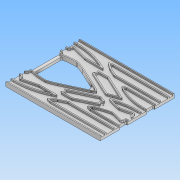
# Autodesk Inventor part: PocketPoint
Saved by Autodesk Inventor 2021 (Build 250183000, 183)
## iProperties
Created: 2021-03-04
Part Number: PocketPoint
Material: 一般
Document SubType Name: Modeling
Designer: kumagai
Density: 1 g/cm^3
Appearance: 既定
Author: kumagai
Autodesk Inventor part; units mm, degrees
ref_plane "YZ Plane" through (0, 0, 0) normal (1, 0, 0) x (0, 1, 0)
ref_plane "XZ Plane" through (0, 0, 0) normal (0, 1, 0) x (-1, 0, 0)
ref_plane "XY Plane" through (0, 0, 0) normal (0, 0, 1) x (1, 0, 0)
sketch "スケッチ1" plane through (0, 0, 0) normal (0, 1, 0) x (-1, 0, 0)
  line L0 (0, -199.2237) -> (0, 200.4653) projected
  line L1 (-205.9572, 0) -> (190.052, 0) projected
  line L2 (92.5, -106.7983) -> (92.5, -71.9832)
  line L3 (-92.5, -104.7638) -> (-92.5, -76.5833)
  line L4 (-113.8272, -72.75) -> (-139.8678, -72.75)
  line L5 (-115.1264, 72.75) -> (-146.0495, 72.75)
  line L6 (-92.5, -72.75) -> (92.5, -72.75)
  line L7 (92.5, -72.75) -> (92.5, -34.75)
  line L8 (-92.5, -34.75) -> (-92.5, -72.75)
  line L9 (-92.5, 72.75) -> (92.5, 72.75)
  line L10 (92.5, 72.75) -> (92.5, 34.75)
  line L11 (-92.5, 34.75) -> (-92.5, 72.75)
  line L12 (128.5967, -53.75) -> (-115.1264, -53.75)
  line L13 (133.4793, 53.75) -> (-123.0769, 53.75)
  line L14 (-117.8804, 0) -> (-149.3845, 0)
  line L15 (92.5, -70.75) -> (-92.5, -70.75)
  line L16 (92.5, 70.75) -> (-92.5, 70.75)
  line L17 (-92.5, -19) -> (-92.5, 19)
  line L18 (-92.5, 19) -> (-90.5855, 19)
  line L19 (-92.5, -19) -> (-87.5, -19)
  line L20 (-92.5, -17) -> (-87.5, -17)
  line L21 (-92.5, 17) -> (-90.5855, 17)
  line L22 (92.5, -63.05) -> (-92.5, -63.05)
  line L23 (92.5, -60.65) -> (-92.5, -60.65)
  line L24 (92.5, -46.85) -> (-92.5, -46.85)
  line L25 (92.5, -44.45) -> (-92.5, -44.45)
  line L26 (-111.5116, -25.1237) -> (108.8826, 77.6478)
  line L27 (-111.5116, 25.1237) -> (108.8826, -77.6478)
  line L28 (-97.9488, -37.5567) -> (-102.497, -39.6775)
  line L29 (-102.6652, -28.6119) -> (-107.2133, -30.7327)
  line L30 (-101.0738, -30.5179) -> (-105.622, -32.6387)
  line L31 (-96.3211, -39.0044) -> (-100.8692, -41.1253)
  line L32 (-108.7666, -16.2304) -> (-113.3147, -18.3512)
  line L33 (-110.4448, -14.3649) -> (-114.993, -16.4857)
  line L34 (-114.1016, -7.574) -> (-118.6498, -9.6949)
  line L35 (-114.2638, -5.4429) -> (-118.8119, -7.5637)
  line L36 (-97.9488, 37.5567) -> (-102.497, 39.6775)
  line L37 (-102.6652, 28.6119) -> (-107.2133, 30.7327)
  line L38 (-101.0738, 30.5179) -> (-105.622, 32.6387)
  line L39 (-96.3211, 39.0044) -> (-100.8692, 41.1253)
  line L40 (-108.7666, 16.2304) -> (-113.3147, 18.3512)
  line L41 (-110.4448, 14.3649) -> (-114.993, 16.4857)
  line L42 (-114.1016, 7.574) -> (-118.6498, 9.6949)
  line L43 (-114.2638, 5.4429) -> (-118.8119, 7.5637)
  line L44 (-5.3544, 3.414) -> (38.5952, 23.9081)
  line L45 (-6.1996, 5.2266) -> (37.75, 25.7207)
  arc A0 (54.8664, 32.1363) -> (37.75, 25.7207) centre (87.5, -80.9685) ccw
  arc A1 (87.5, 60.65) -> (27.6494, 47.3814) centre (87.5, -80.9685) ccw
  arc A2 (87.5, 63.05) -> (26.6351, 49.5566) centre (87.5, -80.9685) ccw
  line L46 (87.5, -11.0193) -> (87.5, 9.6949)
  line L47 (22.0715, 26.9057) -> (-24.3751, 5.2473)
  arc A3 (20.6744, 35.131) -> (22.099, 28.705) centre (24.0122, 32.5) ccw
  line L48 (19.005, 28.1239) -> (-25.3894, 7.4224)
  line L49 (92.5, 34.75) -> (91.5, 34.75)
  arc A4 (17.6247, 34.35) -> (19.005, 28.1239) centre (24.0122, 32.5) ccw
  line L50 (11.7288, 51.1017) -> (-1.4507, 44.9559)
  line L51 (10.7146, 53.2768) -> (-2.465, 47.1311)
  line L52 (-3.7329, 46.85) -> (-92.5, 46.85)
  line L53 (-3.7329, 44.45) -> (-92.5, 44.45)
  line L54 (12.544, 51.5723) -> (23.6088, 59.32)
  line L55 (23.294, 61.105) -> (16.7221, 62.866)
  line L56 (11.1674, 53.5383) -> (19.7729, 59.5639)
  line L57 (92.5, 60.65) -> (87.5, 60.65)
  line L58 (15.3244, 60.65) -> (-92.5, 60.65)
  line L59 (92.5, 63.05) -> (87.5, 63.05)
  line L60 (15.3244, 63.05) -> (-92.5, 63.05)
  line L61 (19.7729, 59.5639) -> (16.1009, 60.5478)
  arc A5 (23.6088, 59.32) -> (23.294, 61.105) centre (23.0352, 60.1391) ccw
  arc A6 (10.7146, 53.2768) -> (11.1674, 53.5383) centre (9.4467, 55.9957) ccw
  arc A7 (16.1009, 60.5478) -> (15.3244, 60.65) centre (15.3244, 57.65) ccw
  arc A8 (11.7288, 51.1017) -> (12.544, 51.5723) centre (9.4467, 55.9957) ccw
  arc A9 (16.7221, 62.866) -> (15.3244, 63.05) centre (15.3244, 57.65) ccw
  arc A10 (-3.7329, 44.45) -> (-1.4507, 44.9559) centre (-3.7329, 49.85) ccw
  arc A11 (-3.7329, 46.85) -> (-2.465, 47.1311) centre (-3.7329, 49.85) ccw
  line L62 (-35.4314, 29.1105) -> (-37.75, 28.0293)
  line L63 (-36.2766, 30.9231) -> (-38.5952, 29.8419)
  line L64 (-37.9474, 36.75) -> (-87.5, 36.75)
  line L65 (17.6247, 34.35) -> (0.3685, 34.35)
  line L66 (-37.9474, 34.75) -> (-87.5, 34.75)
  arc A12 (-63.697, 21.4746) -> (-38.5952, 29.8419) centre (-87.5, 134.7185) ccw
  arc A13 (-63.2856, 19.5173) -> (-37.75, 28.0293) centre (-87.5, 134.7185) ccw
  line L67 (-87.5, 126.6079) -> (-87.5, 142.8291)
  line L68 (26.5097, 46.85) -> (27.6494, 47.3814)
  line L69 (-38.0005, 19.4165) -> (-1.9137, 36.2441)
  line L70 (19.7721, 46.3563) -> (26.6351, 49.5566)
  line L71 (85.7327, 47.3926) -> (84.7595, 51.2358)
  line L72 (83.5446, 51.9597) -> (54.5417, 44.6152)
  line L73 (88.0593, 47.9818) -> (87.086, 51.825)
  line L74 (82.9554, 54.2863) -> (53.9526, 46.9418)
  line L75 (92.5, 46.85) -> (89.5134, 46.85)
  line L76 (53.2161, 46.85) -> (26.5097, 46.85)
  line L77 (92.5, 44.45) -> (89.5134, 44.45)
  line L78 (53.2161, 44.45) -> (20.1947, 44.45)
  line L79 (92.5, 36.75) -> (91.5, 36.75)
  line L80 (19.8891, 36.75) -> (0.3685, 36.75)
  circle A14 centre (24.0122, 32.5) radius 1
  arc A15 (22.0715, 26.9057) -> (22.099, 28.705) centre (21.6489, 27.812) ccw
  arc A16 (20.6744, 35.131) -> (19.8891, 36.75) centre (19.8891, 35.75) ccw
  arc A17 (62.91, 42.0158) -> (40.2524, 35.2101) centre (87.5, -80.9685) ccw
  line L81 (87.5, 32.75) -> (87.5, 30.0175)
  arc A18 (86.2722, 29.0437) -> (56.1923, 32.3319) centre (57.7026, -93.0817) ccw
  arc A19 (85.8166, 27.0963) -> (56.2163, 30.332) centre (57.7026, -93.0817) ccw
  arc A20 (55.4208, 30.2147) -> (38.5952, 23.9081) centre (87.5, -80.9685) ccw
  arc A21 (88.0593, 47.9818) -> (89.5134, 46.85) centre (89.5134, 48.35) ccw
  arc A22 (84.7595, 51.2358) -> (83.5446, 51.9597) centre (83.7901, 50.9903) ccw
  arc A23 (85.7327, 47.3926) -> (89.5134, 44.45) centre (89.5134, 48.35) ccw
  arc A24 (87.086, 51.825) -> (82.9554, 54.2863) centre (83.7901, 50.9903) ccw
  arc A25 (53.2161, 44.45) -> (54.5417, 44.6152) centre (53.2161, 49.85) ccw
  arc A26 (53.2161, 46.85) -> (53.9526, 46.9418) centre (53.2161, 49.85) ccw
  arc A27 (19.7721, 46.3563) -> (20.1947, 44.45) centre (20.1947, 45.45) ccw
  arc A28 (91.5, 34.75) -> (89.5, 32.75) centre (91.5, 32.75) ccw
  arc A29 (91.5, 36.75) -> (87.5, 32.75) centre (91.5, 32.75) ccw
  line L82 (89.5, 32.75) -> (89.5, 30.0175)
  arc A30 (86.2722, 29.0437) -> (87.5, 30.0175) centre (86.5, 30.0175) ccw
  arc A31 (85.8166, 27.0963) -> (89.5, 30.0175) centre (86.5, 30.0175) ccw
  arc A32 (56.2163, 30.332) -> (55.4208, 30.2147) centre (56.2525, 27.3322) ccw
  arc A33 (56.1923, 32.3319) -> (54.8664, 32.1363) centre (56.2525, 27.3322) ccw
  line L83 (-34.6766, 29.5463) -> (-29.7157, 33.02)
  line L84 (-30.0304, 34.805) -> (-36.6533, 36.5796)
  line L85 (-35.8238, 31.1846) -> (-32.6195, 33.4282)
  line L86 (-32.6195, 33.4282) -> (-37.1709, 34.6478)
  arc A34 (-36.2766, 30.9231) -> (-35.8238, 31.1846) centre (-37.5445, 33.642) ccw
  arc A35 (-35.4314, 29.1105) -> (-34.6766, 29.5463) centre (-37.5445, 33.642) ccw
  line L87 (-87.5, 36.75) -> (-92.5, 36.75)
  arc A36 (-36.6533, 36.5796) -> (-37.9474, 36.75) centre (-37.9474, 31.75) ccw
  line L88 (-87.5, 34.75) -> (-92.5, 34.75)
  arc A37 (-37.1709, 34.6478) -> (-37.9474, 34.75) centre (-37.9474, 31.75) ccw
  arc A38 (-29.7157, 33.02) -> (-30.0304, 34.805) centre (-30.2892, 33.8391) ccw
  line L89 (24.6013, -19.5893) -> (0, -8.1176)
  line L90 (22.0715, -26.9057) -> (-24.3751, -5.2473)
  line L91 (19.005, -28.1239) -> (-25.3894, -7.4224)
  arc A39 (-39.1516, 0.942) -> (-62.6685, 7.1431) centre (-87.5, -134.7185) ccw
  arc A40 (-87.5, -6.9) -> (-43.8339, 0) centre (-87.5, 134.7185) ccw
  arc A41 (-117.0028, -6.2788) -> (-116.3471, -6.4144) centre (-87.5, 134.7185) ccw
  line L92 (-92.5, -9.3) -> (-87.5, -9.3)
  line L93 (-92.5, -6.9) -> (-87.5, -6.9)
  arc A42 (-87.5, -9.3) -> (-39.1516, -0.942) centre (-87.5, 134.7185) ccw
  line L94 (-92.5, 6.9) -> (-90.4054, 6.9)
  line L95 (-92.5, 9.3) -> (-90.4054, 9.3)
  arc A43 (-28.7483, 5.1627) -> (-37.3938, 8.4872) centre (-87.5, -134.7185) ccw
  arc A44 (-37.6117, 10.2675) -> (-38.028, 17.6172) centre (-39.9412, 13.8222) ccw
  arc A45 (-34.4994, 10) -> (-34.934, 18.1983) centre (-39.9412, 13.8222) ccw
  line L96 (20.097, -15.2822) -> (0, -5.9108)
  arc A46 (22.099, -28.705) -> (20.6744, -35.131) centre (24.0122, -32.5) ccw
  arc A47 (19.005, -28.1239) -> (17.6247, -34.35) centre (24.0122, -32.5) ccw
  circle A48 centre (24.0122, -32.5) radius 1
  arc A49 (22.099, -28.705) -> (22.0715, -26.9057) centre (21.6489, -27.812) ccw
  arc A50 (19.8891, -36.75) -> (20.6744, -35.131) centre (19.8891, -35.75) ccw
  line L97 (92.5, -36.75) -> (42.3385, -36.75)
  line L98 (92.5, -34.75) -> (42.3385, -34.75)
  line L99 (-78.1824, -36.75) -> (-92.5, -36.75)
  line L100 (-78.1824, -34.75) -> (-92.5, -34.75)
  arc A51 (0.3685, 34.35) -> (-0.8994, 34.0689) centre (0.3685, 31.35) ccw
  arc A52 (0.3685, 36.75) -> (-1.9137, 36.2441) centre (0.3685, 31.35) ccw
  line L101 (-35.4314, -29.1105) -> (-37.75, -28.0293)
  line L102 (-36.2766, -30.9231) -> (-38.5952, -29.8419)
  line L103 (-37.9474, -36.75) -> (-87.5, -36.75)
  line L104 (17.6247, -34.35) -> (0.3685, -34.35)
  line L105 (-37.9474, -34.75) -> (-87.5, -34.75)
  line L106 (19.8891, -36.75) -> (0.3685, -36.75)
  line L107 (-34.6766, -29.5463) -> (-29.7157, -33.02)
  line L108 (-30.0304, -34.805) -> (-36.6533, -36.5796)
  line L109 (-35.8238, -31.1846) -> (-32.6195, -33.4282)
  line L110 (-32.6195, -33.4282) -> (-37.1709, -34.6478)
  arc A53 (-35.8238, -31.1846) -> (-36.2766, -30.9231) centre (-37.5445, -33.642) ccw
  arc A54 (-34.6766, -29.5463) -> (-35.4314, -29.1105) centre (-37.5445, -33.642) ccw
  arc A55 (-37.9474, -36.75) -> (-36.6533, -36.5796) centre (-37.9474, -31.75) ccw
  arc A56 (-37.9474, -34.75) -> (-37.1709, -34.6478) centre (-37.9474, -31.75) ccw
  arc A57 (-30.0304, -34.805) -> (-29.7157, -33.02) centre (-30.2892, -33.8391) ccw
  arc A58 (-0.8994, -34.0689) -> (0.3685, -34.35) centre (0.3685, -31.35) ccw
  arc A59 (-1.9137, -36.2441) -> (0.3685, -36.75) centre (0.3685, -31.35) ccw
  arc A60 (-38.5952, -29.8419) -> (-87.5, -19) centre (-87.5, -134.7185) ccw
  arc A61 (-37.75, -28.0293) -> (-87.5, -17) centre (-87.5, -134.7185) ccw
  arc A62 (-36.065, -8.0153) -> (-28.7483, -5.1627) centre (-87.5, 134.7185) ccw
  line L111 (-1.9137, -36.2441) -> (-48.7506, -14.4036)
  line L112 (-0.8994, -34.0689) -> (-44.6592, -13.6634)
  arc A63 (-35.2514, -10.2732) -> (-27.8189, -7.3754) centre (-87.5, 134.7185) ccw
  arc A64 (-48.667, -12.5565) -> (-48.7506, -14.4036) centre (-48.328, -13.4973) ccw
  arc A65 (-25.3894, -7.4224) -> (-27.8189, -7.3754) centre (-26.6572, -10.1414) ccw
  arc A66 (-24.3751, -5.2473) -> (-28.7483, -5.1627) centre (-26.6572, -10.1414) ccw
  arc A67 (-28.7483, 5.1627) -> (-24.3751, 5.2473) centre (-26.6572, 10.1414) ccw
  line L113 (-34.934, 18.1983) -> (-0.8994, 34.0689)
  arc A68 (-37.6117, 10.2675) -> (-37.3938, 8.4872) centre (-37.0635, 9.4311) ccw
  arc A69 (-38.0005, 19.4165) -> (-38.028, 17.6172) centre (-37.5779, 18.5102) ccw
  arc A70 (-27.8189, 7.3754) -> (-34.4994, 10) centre (-87.5, -134.7185) ccw
  arc A71 (-27.8189, 7.3754) -> (-25.3894, 7.4224) centre (-26.6572, 10.1414) ccw
  arc A72 (-52.3064, 12.8617) -> (-70.3129, 16.0234) centre (-87.5, -134.7185) ccw
  arc A73 (-74.1443, 10.0131) -> (-58.4543, 12.7097) centre (-87.5, 134.7185) ccw
  line L114 (-87.4523, 6.8287) -> (-86.6895, 2.5679)
  line L115 (-39.9412, 13.8222) -> (-87.1898, 5.3626)
  line L116 (-86.992, 23.7251) -> (-87.6188, 19.5542)
  line L117 (-39.9412, 13.8222) -> (-87.4082, 20.9556)
  arc A74 (-64.5674, 7.1366) -> (-85.3887, 1.7956) centre (-37.375, -142.1252) ccw
  arc A75 (-85.6835, 24.524) -> (-65.0909, 19.4711) centre (-45.6063, 143.3669) ccw
  line L118 (-89.8148, 6.4057) -> (-89.0519, 2.145)
  arc A76 (-89.8148, 6.4057) -> (-90.4054, 6.9) centre (-90.4054, 6.3) ccw
  arc A77 (-87.4523, 6.8287) -> (-90.4054, 9.3) centre (-90.4054, 6.3) ccw
  arc A78 (-86.6895, 2.5679) -> (-85.3887, 1.7956) centre (-85.7051, 2.7442) ccw
  arc A79 (-89.0519, 2.145) -> (-84.6292, -0.4811) centre (-85.7051, 2.7442) ccw
  arc A80 (-64.1372, 4.7754) -> (-84.6292, -0.4811) centre (-37.375, -142.1252) ccw
  arc A81 (-43.8339, 0) -> (-63.0823, 4.7791) centre (-87.5, -134.7185) ccw
  arc A82 (-62.6685, 7.1431) -> (-64.5674, 7.1366) centre (-63.5996, 1.824) ccw
  arc A83 (-63.0823, 4.7791) -> (-64.1372, 4.7754) centre (-63.5996, 1.824) ccw
  arc A84 (-39.1516, -0.942) -> (-39.1516, 0.942) centre (-39.4873, 0) ccw
  arc A85 (-85.0444, 26.4192) -> (-64.7801, 21.4468) centre (-45.6063, 143.3669) ccw
  line L119 (-89.5966, 19.8514) -> (-88.9698, 24.0223)
  arc A86 (-90.5855, 19) -> (-89.5966, 19.8514) centre (-90.5855, 20) ccw
  arc A87 (-90.5855, 17) -> (-87.6188, 19.5542) centre (-90.5855, 20) ccw
  arc A88 (-85.0444, 26.4192) -> (-88.9698, 24.0223) centre (-86.0031, 23.5765) ccw
  arc A89 (-85.6835, 24.524) -> (-86.992, 23.7251) centre (-86.0031, 23.5765) ccw
  arc A90 (-64.7801, 21.4468) -> (-63.697, 21.4746) centre (-64.3141, 24.4104) ccw
  arc A91 (-65.0909, 19.4711) -> (-63.2856, 19.5173) centre (-64.3141, 24.4104) ccw
  circle A92 centre (-39.9412, 13.8222) radius 1
  line L120 (-5.8073, 3.1526) -> (-10.3096, 0)
  line L121 (-6.9544, 4.7909) -> (-12.6266, 0.8192)
  line L122 (-10.3096, 0) -> (-13.053, 0)
  arc A93 (-12.6266, 0.8192) -> (-13.053, 0) centre (-12.053, 0) ccw
  arc A94 (-5.3544, 3.414) -> (-5.8073, 3.1526) centre (-4.0866, 0.6951) ccw
  arc A95 (-6.1996, 5.2266) -> (-6.9544, 4.7909) centre (-4.0866, 0.6951) ccw
  line L123 (-35.2514, -10.2732) -> (-44.6592, -13.6634)
  line L124 (-36.065, -8.0153) -> (-48.667, -12.5565)
  point P0 (0, 0)
  point P1 (-87.7021, 19)
  point P2 (0, 26.875)
  point P3 (-41.7373, 17.674)
  point P4 (87.5, 36.75)
  point P5 (25.8083, 28.6482)
  point P6 (24.0122, 36.75)
  point P7 (25.3655, 60.55)
  point P8 (86.4779, 44.45)
  point P9 (87.5, 28.75)
  point P10 (89.5, 26.1747)
  point P11 (-27.959, 34.25)
  point P12 (-37.2891, 36.75)
  point P13 (-27.0869, 6.6308)
  point P14 (-26.5657, 4.2258)
  point P15 (-26.6007, -6.8576)
  point P16 (-87.4651, 6.9)
  point P17 (-12.6758, 0)
  point P18 (25.8083, -28.6482)
  point P19 (24.0122, -36.75)
  point P20 (-27.959, -34.25)
  point P21 (-37.2891, -36.75)
  point P22 (-26.5657, -4.2258)
  point P23 (-26.6007, 6.8576)
  point P24 (-87.8948, 9.3)
  point P25 (-86.4849, 1.4252)
  point P26 (-86.8137, 24.9112)
  point P27 (-88.0026, 17)
  point P28 (-87.7125, 0)
  point P29 (-83.1619, 0)
  dimension "d0" = 185
  dimension "d1" = 145.5
  dimension "d2" = 107.5
  dimension "d5" = 2
  dimension "d6" = 2
  dimension "d7" = 18.6
  dimension "d8" = 2.4
  dimension "d9" = 38
  dimension "d12" = 2
  dimension "d16" = 25
  dimension "d18" = 26.875
  dimension "d19" = 38
  dimension "d20" = 2
  dimension "d23" = 18.6
  dimension "d24" = 2.4
  dimension "d26" = 5
  dimension "d27" = 8.5
  dimension "d29" = 18.6
  dimension "d30" = 2.4
  dimension "d31" = 10
  dimension "d32" = 15
  dimension "d33" = 2.8
  dimension "d34" = 2.5
  dimension "d35" = 1
  dimension "d36" = 3
  dimension "d37" = 3
  dimension "d41" = 3
  dimension "d42" = 38
  dimension "d44" = 5
  dimension "d45" = 2
  dimension "d46" = 2.4
  dimension "d47" = 1
  dimension "d48" = 125.4185
  dimension "d50" = 63.4878
  dimension "d51" = 63.4878
  dimension "d53" = 8
  dimension "d56" = 1.5
  dimension "d57" = 1
  dimension "d62" = 3
  dimension "d64" = 1
  dimension "d65" = 29.7974
  dimension "d66" = 129.8317
  dimension "d71" = 2
  dimension "d74" = 1
  dimension "d75" = 29.7974
  dimension "d77" = 129.8317
  dimension "d78" = 125.4227
  dimension "d79" = 8
  dimension "d84" = 3
  dimension "d86" = 3
  dimension "d87" = 10
  dimension "d88" = 15
  dimension "d89" = 2.5
  dimension "d90" = 1.5
  dimension "d93" = 3
  dimension "d95" = 3
  dimension "d96" = 1
  dimension "d97" = 18.6
  dimension "d98" = 2.4
  dimension "d99" = 8.5
  dimension "d100" = 13.3
  dimension "d102" = 38
  dimension "d103" = 2.4
  dimension "d106" = 3
  constraints: 244 end point, 199 point on circle, 154 tangent, 96 centre point, 83 point on line, 59 symmetric about line, 36 parallel, 29 collinear, 27 coincident, 16 horizontal, 15 perpendicular, 6 vertical, 5 concentric, 2 equal radius, 1 line through centre, 1 vertical alignment, 46 other
  measures "d0" distance between parallel lines of L3 L2
  measures "d1" distance between parallel lines of L5 L4
  measures "d2" distance between parallel lines of L13 L12
  measures "d5" distance between parallel lines of L9 L16
  measures "d6" distance between parallel lines of L6 L15
  measures "d7" distance between parallel lines of L25 L22
  measures "d8" distance between parallel lines of L22 L23
  measures "d9" distance between parallel lines of L18 L19
  measures "d12" distance between parallel lines of L19 L20
  measures "d16" angle of L26 L1
  measures "d18" distance from line of L1 point (0, 26.875)
  measures "d19" distance between parallel lines of L35 L31
  measures "d20" distance between parallel lines of L28 L31
  measures "d23" distance between parallel lines of L33 L30
  measures "d24" distance between parallel lines of L29 L30
  measures "d26" distance between parallel lines of L2 L46
  measures "d27" diameter of A3
  measures "d29" distance between parallel lines of L60 L53
  measures "d30" distance between parallel lines of L60 L58
  measures "d31" angle of L50 L54
  measures "d32" angle of L60 L55
  measures "d33" distance from line of point (25.365, 60.55) L50
  measures "d34" distance from line of point (25.365, 60.55) L60
  measures "d35" radius of A5
  measures "d36" radius of A6
  measures "d37" radius of A7
  measures "d41" radius of A11
  measures "d42" distance between parallel lines of L9 L66
  measures "d45" diameter of A14
  measures "d46" radial gap between concentric circles of A4 A3
  measures "d47" radius of A15
  measures "d48" radius of A17
  measures "d50" distance from line of L81 A3.centre
  measures "d51" distance from line of A3.centre L71
  measures "d53" distance from line of point (86.478, 44.45) L72
  measures "d56" radius of A21
  measures "d57" radius of A22
  measures "d62" radius of A26
  measures "d64" radius of A27
  measures "d65" distance from line of A17.centre L71
  measures "d66" distance from line of A17.centre L72
  measures "d71" radius of A28
  measures "d74" radius of A30
  measures "d75" distance from line of L46 A18.centre
  measures "d77" distance from line of L79 A18.centre
  measures "d78" radius of A18
  measures "d79" distance from line of point (87.5, 28.75) L79
  measures "d84" radius of A32
  measures "d86" radius of A31
  measures "d87" angle of L83 L62
  measures "d88" angle of L64 L84
  measures "d89" vertical distance of point (-27.959, 34.25) point (-37.289, 36.75)
  measures "d90" distance from line of L62 point (-27.959, 34.25)
  measures "d93" radius of A34
  measures "d95" radius of A37
  measures "d96" radius of A38
  measures "d97" distance between parallel lines of L95 L92
  measures "d98" distance between parallel lines of L92 L93
  measures "d99" diameter of A44
  measures "d100" diameter of A45
  measures "d102" distance between parallel lines of L100 L6
  measures "d103" distance between parallel lines of L80 L65
  measures "d106" radius of A51
extrude "Symm" add sketch "スケッチ1" along normal blind 3.2 contours L44 A94 L120 L1 A93 L121 A95 L45 L0 | L0 L45 A0 A33 A18 A30 L81 A29 L79 L10 L49 A28 L82 A31 A19 A32 A20 L44 | L50 A10 L53 L11 L52 A11 L51 L0 | L0 L51 A6 L56 L13 L54 A8 L50 | L78 A27 L70 A2 L13 A1 L68 L76 L26 | L26 L76 A26 L74 L13 A24 L73 A21 L75 L10 L77 A23 L71 A22 L72 A25 L78 | L58 L11 L60 L0 | L0 L60 A9 L55 A5 L54 L13 L56 L61 A7 L58 | L74 A24 L13 | L13 A2 L26 A1 | L26 A2 L59 L10 L57 A1 | L16 L11 L9 L0 | L0 L9 L10 L16
extrude "ASym" add sketch "スケッチ1" along normal blind 3.2 contours L90 A49 A46 A50 L27 L104 A47 L91 L0 | L0 L91 A65 A63 L123 L27 L124 A62 A66 L90 | A58 L104 L27 A50 L106 A59 L0 | L0 A59 L111 A64 L124 L27 L123 L112 A58 | L47 A67 A43 A68 L26 A45 A70 A71 L48 L0 | L0 L48 A4 L65 L26 A16 A3 A15 L47 | A84 A42 L27 A40 L1 | L1 A81 L26 A39 A84 | A42 L26 A40 L27 | A81 A83 A80 L27 A74 A82 A39 L26 | A42 L92 L17 L93 A40 L26 | A51 L113 A45 L26 A68 A44 A69 L69 A52 L0 | L0 A52 L80 A16 L26 L65 A51 | L1 A79 L118 A76 L94 L17 L95 A77 L114 A78 A74 L27 A80 | L8 L100 L105 A56 L110 L109 A53 L102 A60 L19 L17 L20 A61 L101 A54 L107 A57 L108 A55 L103 L99 | L17 L18 A86 L119 A88 A85 A90 A12 L63 A34 L85 L86 A37 L66 L88 L11 L87 L64 A36 L84 A38 L83 A35 L62 A13 A91 A75 A89 L116 A87 L21
mirror "ミラー1" about plane through (0, 0, 0) normal (0, 0, 1) of "Symm"
sketch "スケッチ2" plane through (0, 0, 0) normal (0, 1, 0) x (-1, 0, 0)
  line L0 (92.5, 72.75) -> (-92.5, 72.75) projected
  line L1 (92.5, 72.75) -> (92.5, 34.75) projected
  line L2 (-92.5, 34.75) -> (-92.5, 72.75) projected
  line L3 (-92.5, -19) -> (-92.5, 19) projected
  line L4 (-92.5, -34.75) -> (-92.5, -72.75) projected
  line L5 (92.5, -72.75) -> (-92.5, -72.75) projected
  line L6 (92.5, -72.75) -> (92.5, -34.75) projected
  circle A0 centre (24.0122, 32.5) radius 1 projected
  circle A1 centre (24.0122, -32.5) radius 1 projected
  circle A2 centre (-39.9412, 13.8222) radius 1 projected
  line L7 (-92.5, 34.75) -> (-37.9474, 34.75) projected
  line L8 (-92.5, 34.75) -> (-89.5, 34.75)
  line L9 (-89.5, 34.75) -> (-89.5, 19)
  line L10 (-92.5, 19) -> (-92.5, 17) projected
  line L11 (-89.5, 19) -> (-92.5, 19)
  line L12 (-92.5, -19) -> (-89.5, -19)
  line L13 (-89.5, -19) -> (-89.5, -34.75)
  line L14 (-37.9474, -34.75) -> (-92.5, -34.75) projected
  line L15 (-89.5, -34.75) -> (-92.5, -34.75)
  line L16 (92.5, 34.75) -> (89.5, 34.75)
  line L17 (89.5, 34.75) -> (89.5, -34.75)
  line L18 (89.5, -34.75) -> (92.5, -34.75)
  line L19 (-5.3544, 3.414) -> (38.5952, 23.9081) projected
  line L20 (-5.3544, -3.414) -> (38.5952, -23.9081) projected
  arc A3 (55.4208, 30.2147) -> (38.5952, 23.9081) centre (87.5, -80.9685) ccw projected
  arc A4 (38.5952, -23.9081) -> (55.4208, -30.2147) centre (87.5, 80.9685) ccw projected
  arc A5 (56.2163, -30.332) -> (85.8166, -27.0963) centre (57.7026, 93.0817) ccw projected
  arc A6 (56.2163, 30.332) -> (55.4208, 30.2147) centre (56.2525, 27.3322) ccw projected
  arc A7 (85.8166, 27.0963) -> (56.2163, 30.332) centre (57.7026, -93.0817) ccw projected
  arc A8 (85.8166, 27.0963) -> (56.2163, 30.332) centre (57.7026, -93.0817) ccw projected
  line L21 (83.5, 27.6148) -> (83.5, -27.6148)
  arc A9 (6.76, 9.0631) -> (6.76, -9.0631) centre (10.9862, 0) ccw
  line L22 (-129.5, 0) -> (129.5, 0) projected
  arc A10 (55.4208, -30.2147) -> (56.2163, -30.332) centre (56.2525, -27.3322) ccw projected
  point P0 (0, 0)
  point P1 (-12.6758, 0)
  point P2 (-92.5, 0)
  point P3 (83.5, 0)
  point P4 (89.5, 0)
  point P5 (0.9862, 0)
  dimension "d171" = 3
  dimension "d172" = 3
  dimension "d173" = 6
  dimension "d174" = 10
  constraints: 20 end point, 5 perpendicular, 5 point on line, 4 point on circle, 2 horizontal, 2 vertical, 1 centre point, 1 collinear, 1 tangent
  measures "d171" distance between parallel lines of L9 L3
  measures "d172" distance between parallel lines of L1 L17
  measures "d173" distance between parallel lines of L21 L17
  measures "d174" radius of A9
extrude "Base" add sketch "スケッチ2" against normal blind 5.2 contours L1 L16 L17 L22 L21 A7 A6 A3 L19 A9 L3 L11 L9 L7 L2 L0 | L17 L18 L6 L5 L4 L14 L13 L12 L3 L22 A9 L20 A4 A10 A5 L21
fillet "フィレット1" radius 2 8 edges at (89.5, -2.6, -34.75) (89.5, -2.6, -19) (89.5, -2.6, 19) (89.5, -2.6, 34.75) (-89.5, -2.6, 34.75) (-89.5, -2.6, -34.75) (-83.5, -2.6, 27.6148) (-83.5, -2.6, -27.6148)
sketch "スケッチ3" plane through (0, -5.2, 0) normal (0, -1, 0) x (1, 0, 0)
  circle A0 centre (39.9412, 13.8222) radius 1 projected
  circle A1 centre (-24.0122, 32.5) radius 1 projected
  circle A2 centre (-24.0122, -32.5) radius 1 projected
  line L0 (-24.0122, -30.1329) -> (-21.9622, -31.3164)
  line L1 (-21.9622, -31.3164) -> (-21.9622, -33.6836)
  line L2 (-21.9622, -33.6836) -> (-24.0122, -34.8671)
  line L3 (-24.0122, -34.8671) -> (-26.0622, -33.6836)
  line L4 (-26.0622, -33.6836) -> (-26.0622, -31.3164)
  line L5 (-26.0622, -31.3164) -> (-24.0122, -30.1329)
  line L6 (39.9412, 16.1893) -> (41.9912, 15.0057)
  line L7 (41.9912, 15.0057) -> (41.9912, 12.6386)
  line L8 (41.9912, 12.6386) -> (39.9412, 11.455)
  line L9 (39.9412, 11.455) -> (37.8912, 12.6386)
  line L10 (37.8912, 12.6386) -> (37.8912, 15.0057)
  line L11 (37.8912, 15.0057) -> (39.9412, 16.1893)
  line L12 (-24.0122, 34.8671) -> (-21.9622, 33.6836)
  line L13 (-21.9622, 33.6836) -> (-21.9622, 31.3164)
  line L14 (-21.9622, 31.3164) -> (-24.0122, 30.1329)
  line L15 (-24.0122, 30.1329) -> (-26.0622, 31.3164)
  line L16 (-26.0622, 31.3164) -> (-26.0622, 33.6836)
  line L17 (-26.0622, 33.6836) -> (-24.0122, 34.8671)
  point P0 (0, 0)
  dimension "d189" = 4.1
  dimension "d190" = 4.1
  dimension "d191" = 4.1
  constraints: 36 end point, 3 coincident, 3 vertical, 39 other
  measures "d189" distance between parallel lines of L4 L1
  measures "d190" distance between parallel lines of L7 L10
  measures "d191" distance between parallel lines of L16 L13
extrude "Hex" cut sketch "スケッチ3" against normal blind 2.5 contours A0 | A1 | A2 | L0 L1 L2 L3 L4 L5 | L6 L7 L8 L9 L10 L11 | L12 L13 L14 L15 L16 L17
equation "\"d0\" = StraightLength - 2 * ConnectorLength"
equation "\"d1\" = 0.5 * StraightLength + RailWidth"
equation "\"d2\" = 0.5 * StraightLength"
equation "\"d5\" = OuterWall"
equation "\"d6\" = OuterWall"
equation "\"d7\" = InsideWidth"
equation "\"d8\" = InnerWall"
equation "\"d9\" = RailWidth"
equation "\"d12\" = OuterWall"
equation "\"d18\" = 0.125 * StraightLength"
equation "\"d19\" = RailWidth"
equation "\"d20\" = OuterWall"
equation "\"d23\" = InsideWidth"
equation "\"d24\" = InnerWall"
equation "\"d29\" = InsideWidth"
equation "\"d30\" = InnerWall"
equation "\"d3\" = RailWidth"
equation "\"d4\" = RailWidth"
equation "\"d11\" = InsideWidth"
equation "\"d13\" = InnerWall"
equation "\"d14\" = InsideWidth"
equation "\"d15\" = InnerWall"
equation "\"StraightLength\" = 215"
equation "\"ConnectorLength\" = 15"
equation "\"RailWidth\" = 38"
equation "\"OuterWall\" = 2"
equation "\"InsideWidth\" = 18.6"
equation "\"InnerWall\" = 2.4"
